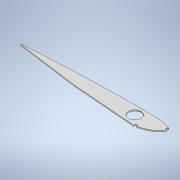
# Autodesk Inventor part: airfoil blueprint
Saved by Autodesk Inventor 2022 (Build 260153000, 153)
## iProperties
Created: 2021-03-06
Part Number: airfoil blueprint
Material: Generic
Document SubType Name: Modeling
Designer: Ferdinand Hubbard
Density: 1 g/cm^3
Appearance: Default
Author: Ferdinand Hubbard
Autodesk Inventor part; units mm, degrees
ref_plane "YZ Plane" through (0, 0, 0) normal (1, 0, 0) x (0, 1, 0)
ref_plane "XZ Plane" through (0, 0, 0) normal (0, 1, 0) x (-1, 0, 0)
ref_plane "XY Plane" through (0, 0, 0) normal (0, 0, 1) x (1, 0, 0)
sketch "Sketch1" plane through (0, 0, 0) normal (0, 1, 0) x (-1, 0, 0)
  spline S0 degree 4 poles (51.979, 34.2431) (49.1051, 33.7566) (39.5332, 31.5872) (30.1137, 28.1904) (19.6059, 22.8943) (13.0923, 18.5073) (7.8605, 14.3051) (3.9363, 9.4088) (1.5106, 6.3896) (0.0434, 1.3996) (-0.032, 0.3871) (0.028, -0.8915) (0.1768, -1.4854) (0.3983, -2.0441) (0.8215, -2.5037) (1.3408, -2.946) (2.6667, -3.7655) (3.7155, -4.2634) (10.6098, -6.747) (15.9249, -7.4764) (25.5133, -9.1262) (35.8155, -9.8616) (48.4495, -10.5455) (62.4279, -10.8762) (77.9663, -11.0677) (94.722, -11.0635) (112.5613, -10.9225) (131.2432, -10.6462) (150.5553, -10.2615) (170.2642, -9.7779) (190.1377, -9.2151) (209.9398, -8.5807) (229.4366, -7.8911) (248.3971, -7.1484) (266.6047, -6.3637) (283.8414, -5.5226) (299.9482, -4.5961) (314.7433, -3.6129) (328.1612, -2.6484) (339.8268, -1.769) (350.012, -1.0496) (357.5866, -0.5225) (364.806, -0.1794) (367.4848, -0.031) (370.1657, -0.0078) (369.9872, 0.0018) knots 0 0 0 0 0 0.056172 0.079777 0.102171 0.123272 0.142974 0.16113 0.176202 0.188392 0.197687 0.204488 0.210696 0.216571 0.223012 0.230232 0.240513 0.254518 0.272366 0.294434 0.318911 0.345468 0.373865 0.403873 0.435249 0.467749 0.501146 0.535218 0.569752 0.604537 0.639365 0.674029 0.708317 0.742021 0.774934 0.806859 0.837599 0.866942 0.894636 0.920358 0.943684 0.964014 0.980302 1 1 1 1 1
  circle A0 centre (370, 0) radius 160 construction
  line L0 (370, 0) -> (211.4974, 21.8387)
  circle A1 centre (211.4974, 21.8387) radius 160 construction
  line L1 (211.4974, 21.8387) -> (51.979, 34.2431)
  line L2 (-0.096, 2.719) -> (4.904, 2.719)
  line L3 (4.904, 2.719) -> (4.904, -2.281)
  line L4 (4.904, -2.281) -> (-0.096, -2.281)
  line L5 (-0.096, -2.281) -> (-0.096, 2.719)
  circle A2 centre (369.9872, 0.0018) radius 3 construction
  line L6 (365.7713, 2.7478) -> (370.7713, 2.7478)
  line L7 (370.7713, 2.7478) -> (370.7713, -2.2522)
  line L8 (370.7713, -2.2522) -> (365.7713, -2.2522)
  line L9 (365.7713, -2.2522) -> (365.7713, 2.7478)
  line L10 (211.4974, 21.8387) -> (210.0997, -8.5616) construction
  line L11 (46.4065, 34.5291) -> (51.4065, 34.5291)
  line L12 (51.4065, 34.5291) -> (51.4065, 29.5291)
  line L13 (51.4065, 29.5291) -> (46.4065, 29.5291)
  line L14 (46.4065, 29.5291) -> (46.4065, 34.5291)
  line L15 (46.4065, 34.5291) -> (51.4065, 29.5291) construction
  line L16 (51.4065, 34.5291) -> (46.4065, 29.5291) construction
  circle A3 centre (72.7388, 10.8459) radius 15.5
  point P0 (0, 0)
  point P1 (370, 0)
  point P2 (35.937, 30.0257)
  point P3 (27.0238, 26.4761)
  point P4 (19.2974, 22.4624)
  point P5 (12.8156, 18.139)
  point P6 (7.6237, 13.6489)
  point P7 (3.7499, 9.1521)
  point P8 (1.2115, 4.8535)
  point P9 (0.0668, 1.0195)
  point P10 (0.0003, -0.0638)
  point P11 (0.0755, -0.9849)
  point P12 (0.2106, -1.5356)
  point P13 (0.4302, -2.0122)
  point P14 (0.7739, -2.4345)
  point P15 (1.2488, -2.8423)
  point P16 (2.1566, -3.4383)
  point P17 (3.2773, -4.0196)
  point P18 (8.2772, -5.8071)
  point P19 (15.3669, -7.4261)
  point P20 (24.3167, -8.7706)
  point P21 (35.0526, -9.7678)
  point P22 (47.5438, -10.4262)
  point P23 (61.6814, -10.8267)
  point P24 (77.2847, -11.0213)
  point P25 (94.162, -11.0379)
  point P26 (112.1091, -10.9014)
  point P27 (130.911, -10.6315)
  point P28 (150.3435, -10.2474)
  point P29 (170.176, -9.7646)
  point P30 (190.1737, -9.1986)
  point P31 (229.7182, -7.8653)
  point P32 (248.7963, -7.1166)
  point P33 (267.1071, -6.3194)
  point P34 (284.4371, -5.4606)
  point P35 (300.619, -4.5258)
  point P36 (315.5184, -3.5432)
  point P37 (328.988, -2.5786)
  point P38 (340.8625, -1.7041)
  point P39 (350.9622, -0.9861)
  point P40 (359.0984, -0.4682)
  point P41 (365.0855, -0.1602)
  point P42 (368.7597, -0.0285)
  point P43 (370, 0)
  point P44 (0.4773, 2.719)
  point P45 (0.6305, -2.281)
  point P46 (365.7713, -0.1283)
  point P47 (368.4073, 0.2194)
  point P48 (48.9065, 32.0291)
  point P49 (112.1091, -11.9485)
  point P50 (365.7713, 0.5826)
  point P51 (51.4065, 34.1414)
  point P52 (46.4065, 33.0501)
  dimension "d5" = 160
  dimension "d8" = 160
  dimension "d17" = 5
  dimension "d18" = 5
  dimension "d25" = 6
  dimension "d26" = 5
  dimension "d27" = 5
  dimension "d36" = 5
  dimension "d37" = 5
  dimension "d50" = 368.7594
  dimension "d62" = 31
  constraints: 34 end point, 6 parallel, 3 horizontal, 3 perpendicular, 2 centre point, 2 midpoint, 1 coincident, 1 point on line, 53 other
  measures "d5" distance of L0.end L0.start
  measures "d8" distance of L0.end L1.end
  measures "d17" distance of L3.end L4.end
  measures "d18" distance of L2.end L3.end
  measures "d25" diameter of A2
  measures "d26" distance of L7.end L8.end
  measures "d27" distance of L6.end L7.end
  measures "d36" distance of L12.end L13.end
  measures "d37" distance of L11.end L12.end
  measures "d50" distance of point (368.76, -0.028) point (0, -0.064)
  measures "d62" diameter of A3
extrude "Extrusion4" add sketch "Sketch1" along normal blind 2.5 contours S0 L4 L3 L2 L14 L13 L12 L1 L0 L9
body "Solid4"
